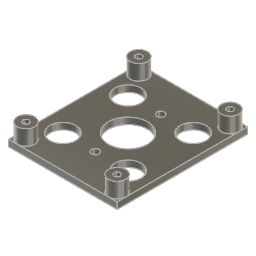
Mosfet Mount (Autodesk Fusion 360 design; units mm, degrees)
Autodesk Fusion 360 part; units mm, degrees
note: some values were not read from the file. Set by a fixed rule: which sketch regions a step uses.
sketch "Sketch1" plane through (0, 0, 0) normal (0, 0, 1) x (1, 0, 0)
  line L0 (21, -26) -> (-21, -26) construction
  line L1 (-21, -26) -> (-21, 26) construction
  line L2 (-21, 26) -> (21, 26) construction
  line L3 (21, 26) -> (21, -26) construction
  line L4 (21, -26) -> (-21, 26) construction
  line L5 (-21, -26) -> (21, 26) construction
  circle A0 centre (-21, 26) radius 1.4
  circle A1 centre (21, 26) radius 1.4
  circle A2 centre (-21, -26) radius 1.4
  circle A3 centre (21, -26) radius 1.4
  line L6 (10, 45) -> (-10, 45) construction
  line L7 (-10, 45) -> (-10, -45) construction
  line L8 (-10, -45) -> (10, -45) construction
  line L9 (10, -45) -> (10, 45) construction
  line L10 (10, 45) -> (-10, -45) construction
  line L11 (-10, 45) -> (10, -45) construction
  circle A4 centre (-10, 45) radius 1.625
  circle A5 centre (10, 45) radius 1.625
  circle A6 centre (21, -26) radius 4
  circle A7 centre (-21, -26) radius 4
  circle A8 centre (-21, 26) radius 4
  circle A9 centre (21, 26) radius 4
  circle A10 centre (-10, 45) radius 4
  circle A11 centre (10, 45) radius 4
  line L12 (25, -26) -> (-25, -26) construction
  line L13 (-25, -26) -> (-25, 26) construction
  line L14 (-25, 26) -> (25, 26) construction
  line L15 (25, 26) -> (25, -26) construction
  line L16 (25, -26) -> (-25, 26) construction
  line L17 (-25, -26) -> (25, 26) construction
  line L18 (21, -30) -> (-21, -30) construction
  line L19 (-21, -30) -> (-21, 30) construction
  line L20 (-21, 30) -> (21, 30) construction
  line L21 (21, 30) -> (21, -30) construction
  line L22 (21, -30) -> (-21, 30) construction
  line L23 (-21, -30) -> (21, 30) construction
  line L24 (25, -30) -> (-25, -30)
  line L25 (-25, -30) -> (-25, 30)
  line L26 (-25, 30) -> (25, 30)
  line L27 (25, 30) -> (25, -30)
  line L28 (-21, 26) -> (21, 26)
  line L29 (21, 26) -> (21, 49.335)
  line L30 (21, 49.335) -> (-21, 49.335)
  line L31 (-21, 49.335) -> (-21, 26)
  dimension "d1" = 52
  dimension "d2" = 42
  dimension "d3" = 2.8
  dimension "d4" = 2.8
  dimension "d5" = 2.8
  dimension "d6" = 2.8
  dimension "d7" = 90
  dimension "d8" = 20
  dimension "d9" = 3.25
  dimension "d10" = 3.25
  dimension "d11" = 8
  dimension "d12" = 8
  dimension "d13" = 8
  dimension "d14" = 8
  dimension "d15" = 8
  dimension "d16" = 8
  dimension "d17" = 60
  dimension "d18" = 50
  constraint perpendicular L0 L1
  constraint parallel L0 L2
  constraint parallel L1 L3
  constraint horizontal L0
  constraint coincident L4 origin
  constraint coincident L5 origin
  constraint coincident L1.end L2.start
  constraint coincident L2.end L3.start
  constraint coincident L0.end L1.start
  constraint coincident L0.start L3.end
  constraint perpendicular L6 L7
  constraint parallel L6 L8
  constraint parallel L7 L9
  constraint horizontal L6
  constraint coincident L10 origin
  constraint coincident L11 origin
  constraint coincident L6.end L7.start
  constraint coincident L6.start L9.end
  constraint concentric A2 A7
  constraint concentric A0 A8
  constraint concentric A4 A10
  constraint concentric A5 A11
  constraint perpendicular L12 L13
  constraint parallel L12 L14
  constraint parallel L13 L15
  constraint horizontal L12
  constraint coincident A6 L12.start
  constraint coincident L16 origin
  constraint coincident L17 origin
  constraint perpendicular L18 L19
  constraint parallel L18 L20
  constraint parallel L19 L21
  constraint horizontal L18
  constraint coincident A6 L18.start
  constraint coincident L22 origin
  constraint coincident L23 origin
  constraint horizontal L24
  constraint vertical L25
  constraint horizontal L26
  constraint vertical L27
  constraint horizontal L28
  constraint vertical L29
  constraint horizontal L30
  constraint vertical L31
  measures "d1" distance of L0.end L1.end
  measures "d2" distance of L1.end L2.end
  measures "d3" diameter of A0
  measures "d4" diameter of A1
  measures "d5" diameter of A2
  measures "d6" diameter of A3
  measures "d7" distance of L6.end L7.end
  measures "d8" distance of L7.end L8.end
  measures "d9" diameter of A4
  measures "d10" diameter of A5
  measures "d11" diameter of A6
  measures "d12" diameter of A7
  measures "d13" diameter of A8
  measures "d14" diameter of A9
  measures "d15" diameter of A10
  measures "d16" diameter of A11
  measures "d17" distance of L24.start L26.end
  measures "d18" distance of L24.start L24.end
extrude "Extrude1" add sketch "Sketch1" along normal blind 3 contours A6 A7 A8 A9 L24 L25 L27 L28 | A8 A9 L26 L28 | A8 L25 L26 | A9 L26 L27 | A7 L24 L25 | A6 L24 L27
extrude "Extrude2" add sketch "Sketch1" along normal blind 10 contours A0 A8 L28 L31 | A0 A8 L28 L31 | A1 A9 L28 L29 | A1 A9 L28 L29 | A7 | A6
sketch "Sketch2" plane through (0, 0, 3) normal (0, 0, 1) x (-1, 0, 0)
  line L0 (25, -26) -> (25, 26)
  line L1 (21, 30) -> (-21, 30)
  line L2 (-25, 26) -> (-25, -26)
  circle A0 centre (0, -15) radius 1.75
  circle A1 centre (0.0425, 15) radius 1.75
  line L3 (-21, -30) -> (21, -30)
  circle A2 centre (0, 0) radius 9
  circle A3 centre (15, -15) radius 6
  circle A4 centre (-15, -15) radius 6
  circle A5 centre (-15, 15) radius 6
  circle A6 centre (15, 15) radius 6
  arc A7 (-21, -30) -> (-25, -26) centre (-21, -26) ccw
  arc A8 (25, -26) -> (21, -30) centre (21, -26) ccw
  arc A9 (21, 30) -> (25, 26) centre (21, 26) ccw
  arc A10 (-25, 26) -> (-21, 30) centre (-21, 26) ccw
  dimension "d23" = 3.5
  dimension "d24" = 3.5
  dimension "d25" = 15
  dimension "d26" = 15
  dimension "d29" = 18
  dimension "d30" = 12
  dimension "d31" = 12
  dimension "d32" = 12
  dimension "d33" = 12
  dimension "d34" = 10
  dimension "d35" = 10
  dimension "d36" = 10
  dimension "d37" = 10
  dimension "d38" = 15
  dimension "d39" = 15
  dimension "d40" = 15
  dimension "d41" = 15
  constraint coincident A2.centre origin
  measures "d23" diameter of A0
  measures "d24" diameter of A1
  measures "d25" vertical distance of A2.centre A1.centre
  measures "d26" distance of A2.centre A0.centre
  measures "d29" diameter of A2
  measures "d30" diameter of A3
  measures "d31" diameter of A4
  measures "d32" diameter of A5
  measures "d33" diameter of A6
  measures "d34" distance of L0 A6.centre
  measures "d35" distance of L0 A3.centre
  measures "d36" distance of L2 A4.centre
  measures "d37" distance of L2 A5.centre
  measures "d38" distance of L1 A6.centre
  measures "d39" distance of L1 A5.centre
  measures "d40" distance of L3 A4.centre
  measures "d41" distance of L3 A3.centre
extrude "Extrude3" cut sketch "Sketch2" against normal blind 9 contours A0 | A1 | A2 | A3 | A4 | A5 | A6
equation "d35 = d34"
equation "d36 = d34"
equation "d37 = d34"
equation "d39 = d38"
equation "d40 = d38"
equation "d41 = d38"
